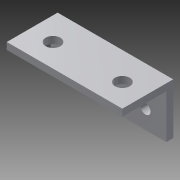
# Autodesk Inventor part: Servo catch
Saved by Autodesk Inventor 2015 (Build 190159000, 159)
## iProperties
Created: 2015-05-18
Part Number: Servo catch
Material: アルミニウム 1100-H14
Document SubType Name: Modeling
Designer: kenta
Density: 2.7 g/cm^3
Appearance: サテン
Mass: 1.97969 g
Surface Area: 11.6502 cm^2
Volume: 0.733219 cm^3
Author: kenta
Autodesk Inventor part; units mm, degrees
ref_plane "YZ Plane" through (0, 0, 0) normal (1, 0, 0) x (0, 1, 0)
ref_plane "XZ Plane" through (0, 0, 0) normal (0, 1, 0) x (-1, 0, 0)
ref_plane "XY Plane" through (0, 0, 0) normal (0, 0, 1) x (1, 0, 0)
sketch "スケッチ1" plane through (0, 0, 0) normal (0, 0, 1) x (1, 0, 0)
  line L0 (-12.5, 5) -> (12.5, 5)
  line L1 (12.5, 5) -> (12.5, -5)
  line L2 (12.5, -5) -> (-12.5, -5)
  line L3 (-12.5, -5) -> (-12.5, 5)
  line L4 (-12.5, 5) -> (12.5, -5) construction
  line L5 (12.5, 5) -> (-12.5, -5) construction
  point P0 (0, 0)
  dimension "d0" = 25
  dimension "d1" = 10
  constraints: 12 end point, 2 midpoint, 2 parallel, 1 horizontal, 1 perpendicular
  measures "d0" distance of L1.end L2.end
  measures "d1" distance of L0.end L1.end
extrude "押し出し1" add sketch "スケッチ1" along normal blind 1
sketch "スケッチ3" plane through (0, 0, 1) normal (0, 0, 1) x (1, 0, 0)
  line L0 (-12.5, 5) -> (12.5, 5)
  line L1 (12.5, 5) -> (12.5, 6)
  line L2 (12.5, 6) -> (-12.5, 6)
  line L3 (-12.5, 6) -> (-12.5, 5)
  point P0 (0, 0)
  dimension "d15" = 25
  dimension "d16" = 1
  constraints: 8 end point, 2 parallel, 1 horizontal, 1 perpendicular
  measures "d15" distance of L2.end L1.end
  measures "d16" distance of L1.end L0.end
extrude "押し出し2" add sketch "スケッチ3" against normal blind 11
sketch "スケッチ7" plane through (0, 0, 0) normal (0, 0, -1) x (-1, 0, 0)
  line L0 (12.5, -5) -> (-12.5, -5)
  line L1 (-12.5, -5) -> (-12.5, 5)
  line L2 (-12.5, 5) -> (12.5, 5)
  line L3 (12.5, 5) -> (12.5, -5)
  point P0 (0, 0)
  constraints: 8 end point, 2 parallel, 1 horizontal, 1 perpendicular
extrude "押し出し4" add sketch "スケッチ7" along normal blind 0.5
sketch "スケッチ8" plane through (-12.5, 5, -10) normal (0, -1, 0) x (1, 0, 0)
  line L0 (0, 0) -> (25, 0)
  line L1 (25, 0) -> (25, 9.5)
  line L2 (25, 9.5) -> (0, 9.5)
  line L3 (0, 9.5) -> (0, 0)
  point P0 (12.5, 10)
  constraints: 8 end point, 2 parallel, 1 horizontal, 1 perpendicular
extrude "押し出し5" add sketch "スケッチ8" along normal blind 0.5
sketch "スケッチ9" plane through (0, 0, 1) normal (0, 0, 1) x (1, 0, 0)
  line L0 (-12.5, 4.5) -> (12.5, 4.5) projected
  line L1 (12.5, -5) -> (12.5, 6) projected
  line L2 (-12.5, 6) -> (-12.5, -5) projected
  point P0 (0, 0)
  point P1 (7.5, 0)
  point P2 (-7.5, 0)
  dimension "d38" = 4.5
  dimension "d39" = 5
  dimension "d40" = 5
  dimension "d41" = 4.5
  measures "d38" distance from line of L0 point (7.5, 0)
  measures "d39" distance from line of L1 point (7.5, 0)
  measures "d40" distance from line of point (-7.5, 0) L2
  measures "d41" distance from line of L0 point (-7.5, 0)
hole "穴3" at (7.5, 0, 1) at (-7.5, 0, 1) direction (0, 0, -1) diameter 3.2 depth 8 tip angle 118
sketch "スケッチ10" plane through (-12.5, 6, 1) normal (0, 1, 0) x (1, 0, 0)
  line L0 (0, 11) -> (25, 11) projected
  line L1 (25, 0) -> (25, 11) projected
  point P0 (12.5, 1)
  point P1 (4.5, 7)
  point P2 (20.5, 7)
  dimension "d49" = 4
  dimension "d50" = 4.5
  dimension "d51" = 4
  dimension "d52" = 16
  measures "d49" distance from line of point (20.5, 7) L0
  measures "d50" distance from line of point (20.5, 7) L1
  measures "d51" distance from line of point (4.5, 7) L0
  measures "d52" distance of point (4.5, 7) point (20.5, 7)
hole "穴4" at (-8, 6, -6) at (8, 6, -6) direction (0, -1, 0) diameter 2.2 depth 8 tip angle 118
